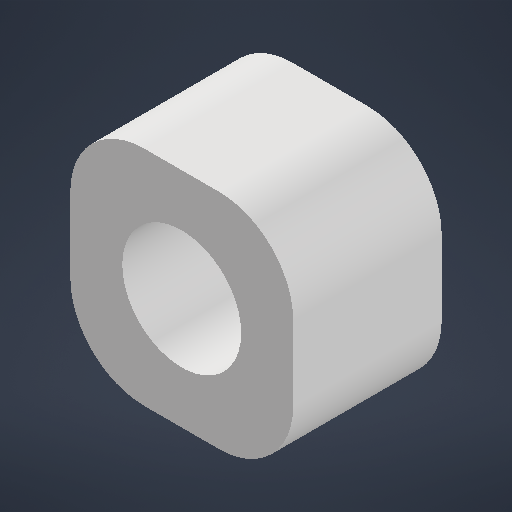
# Autodesk Inventor part: TapónEje
Saved by Autodesk Inventor 2026.2 (Build 302298010, 298A)
## iProperties
Created: 2026-04-17
Part Number: TapónEje
Material: Genérico
Document SubType Name: Modeling
Designer: Jose Carlos
Density: 1 g/cm^3
Appearance: Valor por defecto
Author: Jose Carlos
Autodesk Inventor part; units mm, degrees
ref_plane "YZ Plane" through (0, 0, 0) normal (1, 0, 0) x (0, 1, 0)
ref_plane "XZ Plane" through (0, 0, 0) normal (0, 1, 0) x (-1, 0, 0)
ref_plane "XY Plane" through (0, 0, 0) normal (0, 0, 1) x (1, 0, 0)
sketch "Boceto1" plane through (0, 0, 0) normal (0, 0, 1) x (1, 0, 0)
  circle A0 centre (0, 0) radius 1.4 construction
  circle A1 centre (0, 0) radius 1.6
  line L0 (-3, 3) -> (3, 3)
  line L1 (3, 3) -> (3, -3)
  line L2 (3, -3) -> (-3, -3)
  line L3 (-3, -3) -> (-3, 3)
  line L4 (-3, 3) -> (3, -3) construction
  line L5 (3, 3) -> (-3, -3) construction
  point P0 (0, 0)
  point P1 (0, -3)
  dimension "d0" = 0.2
  dimension "d1" = 3
  dimension "d2" = 3
  constraints: 12 end point, 3 midpoint, 2 parallel, 1 centre point, 1 coincident, 1 horizontal, 1 perpendicular
  measures "d0" radial gap between concentric circles of A0 A1
  measures "d1" distance of A1.centre point (0, -3)
  measures "d2" distance from line of point (0, 0) L1
extrude "Extrusión1" add sketch "Boceto1" against normal blind 4
fillet "Empalme1" radius 2 4 edges at (3, -3, -2) (-3, -3, -2) (-3, 3, -2) (3, 3, -2)
